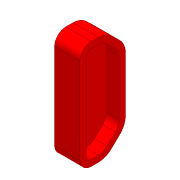
# Autodesk Inventor part: Power_Cap
Saved by Autodesk Inventor 2021.3 (Build 253353000, 353)
## iProperties
Part Number: Power_Cap
Material: PA 6.6
Document SubType Name: Modeling
Designer: SRORF
Mass: 0.0432009 g
Surface Area: 1.17203 cm^2
Volume: 0.0378955 cm^3
Density: 1.14 g/cm^3
Appearance: - 1 Rot
ROT_Density: 1.0
PDB_Ident_Ver: =<PDB_Ident> <PDB_Version>
ROT_Weight: 0.043 g
ROT_Weight_Num: 4.320089905745452e-05
Author: SRORF
Autodesk Inventor part; units mm, degrees
ref_plane "YZ Plane" through (0, 0, 0) normal (1, 0, 0) x (0, 1, 0)
ref_plane "XZ Plane" through (0, 0, 0) normal (0, 1, 0) x (-1, 0, 0)
ref_plane "XY Plane" through (0, 0, 0) normal (0, 0, 1) x (1, 0, 0)
sketch "Skizze2" plane through (0, 0, 0) normal (1, 0, 0) x (0, 1, 0)
  arc A0 (0.4, 7.55) -> (0, 7.15) centre (0.4, 7.15) ccw projected
  line L0 (0.4, 7.55) -> (0.9477, 7.55) projected
  arc A1 (1.6402, 7.2714) -> (0.9477, 7.55) centre (0.9477, 6.55) ccw projected
  line L1 (1.6402, 7.2714) -> (2.2925, 6.6452) projected
  arc A2 (2.6, 5.9238) -> (2.2925, 6.6452) centre (1.6, 5.9238) ccw projected
  line L2 (2.6, 5.9238) -> (2.6, 1.6262) projected
  arc A3 (2.2925, 0.9048) -> (2.6, 1.6262) centre (1.6, 1.6262) ccw projected
  line L3 (2.2925, 0.9048) -> (1.6402, 0.2786) projected
  arc A4 (0.9477, 0) -> (1.6402, 0.2786) centre (0.9477, 1) ccw projected
  line L4 (0.9477, 0) -> (0.4, 0) projected
  arc A5 (0, 0.4) -> (0.4, 0) centre (0.4, 0.4) ccw projected
  line L5 (0, 0.4) -> (0, 7.15) projected
  line L6 (0.9477, 8.05) -> (0.4, 8.05)
  arc A6 (0.4, 8.05) -> (-0.5, 7.15) centre (0.4, 7.15) ccw
  line L7 (-0.5, 7.15) -> (-0.5, 0.4)
  arc A7 (-0.5, 0.4) -> (0.4, -0.5) centre (0.4, 0.4) ccw
  line L8 (0.4, -0.5) -> (0.9477, -0.5)
  arc A8 (0.9477, -0.5) -> (1.9865, -0.0821) centre (0.9477, 1) ccw
  line L9 (1.9865, -0.0821) -> (2.6388, 0.5441)
  arc A9 (2.6388, 0.5441) -> (3.1, 1.6262) centre (1.6, 1.6262) ccw
  line L10 (3.1, 1.6262) -> (3.1, 5.9238)
  arc A10 (3.1, 5.9238) -> (2.6388, 7.0059) centre (1.6, 5.9238) ccw
  line L11 (2.6388, 7.0059) -> (1.9865, 7.6321)
  arc A11 (1.9865, 7.6321) -> (0.9477, 8.05) centre (0.9477, 6.55) ccw
  point P0 (0, 0)
  dimension "d0" = 0.5
  constraints: 12 end point, 12 point on circle, 6 centre point, 11 other
  measures "d0" distance between parallel lines of L7 L5
extrude "Extrusion1" add sketch "Skizze2" along normal blind 1
extrude "Extrusion2" add sketch "Skizze2" against normal blind 1 contours L0 A1 L1 A2 L2 A3 L3 A4 L4 A5 L5 A0 | A11 L11 A10 L10 A9 L9 A8 L8 A7 L7 A6 L6
